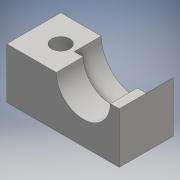
# Autodesk Inventor part: Holder_Mirrored
Saved by Autodesk Inventor 2016 (Build 200138000, 138)
## iProperties
Created: 2015-11-04
Part Number: Holder_Mirrored
Material: Generic
Document SubType Name: Modeling
Designer: PowerStation9000
Density: 1 g/cm^3
Appearance: Default
Author: PowerStation9000
Autodesk Inventor part; units mm, degrees
ref_plane "YZ Plane" through (0, 0, 0) normal (1, 0, 0) x (0, 1, 0)
ref_plane "XZ Plane" through (0, 0, 0) normal (0, 1, 0) x (-1, 0, 0)
ref_plane "XY Plane" through (0, 0, 0) normal (0, 0, 1) x (1, 0, 0)
sketch "Sketch1" plane through (0, 0, 0) normal (0, 1, 0) x (-1, 0, 0)
  arc A0 (-6, 0) -> (6, 0) centre (0, 0) ccw
  arc A1 (-8, 0) -> (8, 0) centre (0, 0) ccw
  line L0 (-17, 0) -> (-17, -11.2563)
  line L1 (-17, -11.2563) -> (8, -11.2563)
  line L2 (8, -11.2563) -> (8, 0)
  line L3 (8, 0) -> (6, 0)
  line L4 (-6, 0) -> (-17, 0)
  line L5 (6, 0) -> (-6, 0) construction
  dimension "d0" = 12
  dimension "d1" = 16
  dimension "d2" = 8
  dimension "d3" = 9
  constraints: 12 end point, 5 point on circle, 4 perpendicular, 2 centre point, 2 coincident, 2 point on line, 1 horizontal, 1 midpoint, 1 vertical
  measures "d0" diameter of A0
  measures "d1" diameter of A1
  measures "d2" distance from line of point (0, 0) L2
  measures "d3" distance from line of A1.start L0
extrude "Tykkelse" add sketch "Sketch1" along normal mid plane 12 contours A1 L2 L1 L0 L4
extrude "Lille cirkel" add sketch "Sketch1" against normal blind 6 contours A0 L3 A1 L4
sketch "Sketch2" plane through (17, 6, -11.2563) normal (0, 0, -1) x (-1, 0, 0)
  circle A0 centre (6, -6) radius 2
  line L0 (0, 0) -> (0, -12) projected
  line L1 (25, -12) -> (0, -12) projected
  point P0 (17, -6)
  dimension "d9" = 4
  dimension "d10" = 6
  dimension "d11" = 6
  constraints: 1 centre point
  measures "d9" diameter of A0
  measures "d10" distance from line of L0 A0.centre
  measures "d11" distance from line of L1 A0.centre
extrude "Monteringshul" cut sketch "Sketch2" against normal up to surface (11.2563 mm away)
mirror "Mirror1" about plane through (17, 0, 0) normal (1, 0, 0) remove original yes
body "Solid1"
